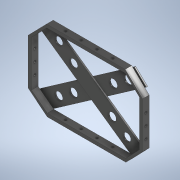
# Autodesk Inventor part: New Chassis
Saved by Autodesk Inventor 2020 (Build 240168000, 168)
## iProperties
Created: 2022-07-18
Part Number: New Chassis
Material: Generic
Document SubType Name: Modeling
Designer: karimi2
Density: 1 g/cm^3
Appearance: Dark Gray
Author: karimi2
Autodesk Inventor part; units mm, degrees
ref_plane "YZ Plane" through (0, 0, 0) normal (1, 0, 0) x (0, 1, 0)
ref_plane "XZ Plane" through (0, 0, 0) normal (0, 1, 0) x (-1, 0, 0)
ref_plane "XY Plane" through (0, 0, 0) normal (0, 0, 1) x (1, 0, 0)
sketch "Sketch1" plane through (0, 0, 0) normal (0, 0, 1) x (1, 0, 0)
  line L0 (0, 0) -> (-116.4534, 0)
  line L1 (-175, 47) -> (-175, 187)
  line L2 (-118.5466, 245) -> (0, 245)
  line L3 (0, 245) -> (0, 0) construction
  line L4 (-118.5466, 235) -> (-9, 235)
  line L5 (-9, 10) -> (-116.4534, 10)
  line L6 (-165, 47) -> (-165, 187)
  line L7 (0, 0) -> (123.5466, 0)
  line L8 (175, 53.5466) -> (175, 193.5466)
  line L9 (121.4534, 245) -> (0, 245)
  line L10 (121.4534, 235) -> (9, 235)
  line L11 (9, 10) -> (123.5466, 10)
  line L12 (165, 53.5466) -> (165, 193.5466)
  line L13 (-9, 235) -> (9, 235)
  line L14 (-9, 10) -> (9, 10)
  line L15 (-175, 187) -> (-118.5466, 245)
  line L16 (-175, 47) -> (-116.4534, 0)
  line L17 (121.4534, 245) -> (175, 193.5466)
  line L18 (175, 53.5466) -> (123.5466, 0)
  line L19 (-175, 47) -> (-165, 47)
  line L20 (-116.4534, 10) -> (-116.4534, 0)
  line L21 (-118.5466, 245) -> (-118.5466, 235)
  line L22 (-175, 187) -> (-165, 187)
  line L23 (-118.5466, 235) -> (-165, 187)
  line L24 (-165, 47) -> (-116.4534, 10)
  line L25 (121.4534, 245) -> (121.4534, 235)
  line L26 (175, 193.5466) -> (165, 193.5466)
  line L27 (121.4534, 235) -> (165, 193.5466)
  line L28 (175, 53.5466) -> (165, 53.5466)
  line L29 (123.5466, 0) -> (123.5466, 10)
  line L30 (123.5466, 10) -> (165, 53.5466)
  point P0 (-175, 245)
  point P1 (-175, 0)
  point P2 (-165, 235)
  point P3 (-165, 10)
  point P4 (175, 245)
  point P5 (175, 0)
  point P6 (165, 235)
  point P7 (165, 10)
  dimension "d0" = 245
  dimension "d1" = 175
  dimension "d4" = 10
  dimension "d7" = 240
  dimension "d9" = 240
  dimension "d10" = 140
  dimension "d12" = 136.142
  dimension "d13" = 133.589
  dimension "d14" = 52.687
  dimension "d15" = 44.062
  dimension "d16" = 44.226
  dimension "d17" = 51.243
  dimension "d18" = 10
  dimension "d19" = 53.5466
  dimension "d20" = 175
  dimension "d21" = 0
  dimension "d22" = 0
  dimension "d23" = 10
  dimension "d24" = 41.4534
  dimension "d25" = 10
  dimension "d26" = 183.5465
  dimension "d27" = 166
  dimension "d28" = 166
  constraints: 62 end point, 11 parallel, 10 perpendicular, 6 symmetric about line, 3 horizontal, 1 horizontal alignment, 1 vertical alignment
  measures "d0" distance of point (-175, 0) point (-175, 245)
  measures "d1" distance of point (-175, 245) L2.end
  measures "d4" distance between parallel lines of L0 L5
  measures "d7" distance of L2.start L9.start
  measures "d9" distance of L0.end L7.end
  measures "d10" distance of L8.end L8.start
  measures "d12" angle of L8 L18
  measures "d13" angle of L27 L8
  measures "d14" angle of L24 L8
  measures "d15" angle of L23 L8
  measures "d16" angle of L15 L8
  measures "d17" angle of L16 L8
  measures "d18" distance between parallel lines of L12 L8
  measures "d19" distance between parallel lines of L25 L8
  measures "d20" distance between parallel lines of L3 L8
  measures "d21" distance from line of point (175, 245) L8
  measures "d22" distance from line of point (175, 0) L8
  measures "d23" distance from line of point (165, 235) L8
  measures "d24" distance from line of point (165, 235) L26
  measures "d25" distance from line of point (165, 10) L8
  measures "d26" distance from line of point (165, 10) L26
  measures "d27" distance from line of L10.end L8
  measures "d28" distance from line of L11.start L8
extrude "Extrusion1" add sketch "Sketch1" along normal blind 20 contours L0 L20 L5 L14 L11 L29 L7 | L16 L19 L24 L20 | L29 L30 L28 L18 | L1 L22 L6 L19 | L28 L12 L26 L8 | L15 L21 L23 L22 | L26 L27 L25 L17 | L2 L9 L25 L10 L13 L4 L21
ref_plane "Work Plane1" through (0, 0, 0) normal (0, 0, -1) x (-1, 0, 0)
sketch "Sketch2" plane through (0, 0, 0) normal (0, 0, -1) x (-1, 0, 0)
  line L0 (-123.5466, 0) -> (-175, 53.5466) projected
  line L1 (-175, 53.5466) -> (-175, 0)
  line L2 (-175, 0) -> (-123.5466, 0)
  line L3 (175, 187) -> (175, 47) projected
  line L4 (175, 47) -> (175, 0)
  line L5 (116.4534, 0) -> (-123.5466, 0) projected
  line L6 (175, 0) -> (116.4534, 0)
  line L7 (-121.4534, 245) -> (118.5466, 245) projected
  line L8 (118.5466, 245) -> (175, 245)
  line L9 (175, 245) -> (175, 187)
  line L10 (-121.4534, 245) -> (-175, 245)
  line L11 (-175, 245) -> (-175, 193.5466)
  line L12 (-175, 193.5466) -> (-121.4534, 245) projected
  line L13 (-160.5333, -20.6513) -> (189.4198, 224.4003)
  line L14 (-189.2819, 20.4027) -> (160.7181, 265.4027)
  circle A0 centre (101, 198.51) radius 12
  circle A1 centre (56, 161.7) radius 12.5
  circle A2 centre (-107.0481, 47.7774) radius 12
  circle A3 centre (-62.0481, 79.2774) radius 12.5
  line L15 (160.7181, 265.4027) -> (189.4198, 224.4003)
  line L16 (-189.238, 20.3554) -> (-160.5333, -20.6513)
  line L17 (118.5466, 245) -> (175, 187) projected
  point P0 (0, 0)
  point P1 (159.1963, 203.2366)
  point P2 (123.8247, 239.5773)
  point P3 (-161.7026, 39.7082)
  point P4 (-126.5613, 3.1373)
  dimension "d32" = 45
  dimension "d33" = 45
  dimension "d34" = 24
  dimension "d35" = 25
  dimension "d36" = 24
  dimension "d37" = 25
  dimension "d38" = 45
  constraints: 25 end point, 4 centre point, 4 perpendicular, 2 vertical, 1 horizontal, 1 parallel, 1 point on line
  measures "d32" horizontal distance of A1.centre A0.centre
  measures "d33" horizontal distance of A2.centre A3.centre
  measures "d34" diameter of A0
  measures "d35" diameter of A1
  measures "d36" diameter of A2
  measures "d37" diameter of A3
  measures "d38" distance from line of A2.centre L0
extrude "Extrusion2" add sketch "Sketch2" along normal blind 4 contours L0 L14 L17 L13
ref_plane "Work Plane3" through (0, 0, -4) normal (0, 0, -1) x (-1, 0, 0)
sketch "Sketch4" plane through (0, 0, -4) normal (0, 0, -1) x (-1, 0, 0)
  line L0 (175, 47) -> (116.4534, 0) projected
  line L1 (116.4534, 0) -> (175, 0)
  line L2 (175, 0) -> (175, 47)
  line L3 (175, 187) -> (175, 245)
  line L4 (118.5466, 245) -> (175, 187) projected
  line L5 (175, 245) -> (118.5466, 245)
  line L6 (-175, 193.5466) -> (-121.4534, 245) projected
  line L7 (-121.4534, 245) -> (-175, 245)
  line L8 (-175, 245) -> (-175, 193.5466)
  line L9 (-123.5466, 0) -> (-175, 0)
  line L10 (-175, 0) -> (-175, 53.5466)
  line L11 (175, 0) -> (-175, 245)
  line L12 (160.906, -20.1342) -> (-189.094, 224.8658)
  line L13 (189.2349, 20.3356) -> (-160.7651, 265.3356)
  line L14 (160.906, -20.1342) -> (189.2349, 20.3356)
  line L15 (-189.094, 224.8658) -> (-160.7651, 265.3356)
  circle A0 centre (105.3249, 48.7726) radius 12
  circle A1 centre (60.3249, 80.2726) radius 12.5
  circle A2 centre (-106.4463, 197.0124) radius 12.5
  circle A3 centre (-61.4463, 165.5124) radius 12.5
  point P0 (0, 0)
  point P1 (163.8873, 38.0789)
  point P2 (-125.7779, 240.8446)
  point P3 (-162.0833, 205.9583)
  point P4 (123.7616, 5.8669)
  dimension "d46" = 24.577
  dimension "d47" = 24.8227
  dimension "d48" = 45
  dimension "d50" = 45
  dimension "d51" = 45
  dimension "d52" = 45
  dimension "d55" = 25
  dimension "d56" = 25
  dimension "d59" = 25
  dimension "d60" = 24
  constraints: 27 end point, 4 centre point, 4 perpendicular, 4 point on line, 3 horizontal, 3 parallel, 1 vertical
  measures "d46" distance between parallel lines of L11 L12
  measures "d47" distance between parallel lines of L11 L13
  measures "d48" horizontal distance of A1.centre A0.centre
  measures "d50" distance from line of L0 A0.centre
  measures "d51" distance from line of A2.centre L6
  measures "d52" horizontal distance of A3.centre A2.centre
  measures "d55" diameter of A3
  measures "d56" diameter of A2
  measures "d59" diameter of A1
  measures "d60" diameter of A0
extrude "Extrusion3" add sketch "Sketch4" along normal blind 4 contours L0 L11 A0 A1 A3 A2 L6 L13 | L0 L12 L6 L11 A2 A3 A1 A0
sketch "Sketch5" plane through (-118.5466, 245, 0) normal (0, 1, 0) x (1, 0, 0)
  line L0 (240, 0) -> (0, 0) projected
  line L1 (0, 0) -> (0, -20) projected
  point P0 (118.5466, 0)
  point P1 (48, -10)
  point P2 (96, -10)
  point P3 (144, -10)
  point P4 (192, -10)
  dimension "d70" = 10
  dimension "d71" = 48
  dimension "d72" = 48
  dimension "d73" = 48
  dimension "d74" = 48
  constraints: 3 horizontal alignment
  measures "d70" distance from line of L0 point (48, -10)
  measures "d71" distance from line of L1 point (48, -10)
  measures "d72" distance of point (96, -10) point (48, -10)
  measures "d73" distance of point (144, -10) point (96, -10)
  measures "d74" distance of point (192, -10) point (144, -10)
hole "Hole1" at (-70.5466, 245, 10) at (-22.5466, 245, 10) at (25.4534, 245, 10) at (73.4534, 245, 10) direction (0, -1, 0) diameter 8 end through all
sketch "Sketch6" plane through (-175, 47, 0) normal (-1, 0, 0) x (0, 0, 1)
  line L0 (0, 0) -> (20, 0) projected
  line L1 (0, 140) -> (0, 0) projected
  point P0 (0, -47)
  point P1 (10, 35)
  point P2 (10, 70)
  point P3 (10, 105)
  dimension "d82" = 35
  dimension "d83" = 10
  dimension "d84" = 35
  dimension "d85" = 35
  constraints: 2 vertical alignment
  measures "d82" distance from line of point (10, 35) L0
  measures "d83" distance from line of L1 point (10, 35)
  measures "d84" distance of point (10, 70) point (10, 35)
  measures "d85" distance of point (10, 105) point (10, 70)
hole "Hole2" at (-175, 82, 10) at (-175, 117, 10) at (-175, 152, 10) direction (1, 0, 0) diameter 8 end through all
body "Solid1"
